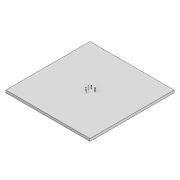
# Autodesk Inventor part: verify_geometry
Saved by Autodesk Inventor 2021 (Build 250183000, 183)
## iProperties
Created: 2022-05-26
Part Number: verify_geometry
Material: Generic
Document SubType Name: Modeling
Designer: Derm
Density: 1 g/cm^3
Appearance: Default
Author: Derm
Autodesk Inventor part; units mm, degrees
ref_plane "YZ Plane" through (0, 0, 0) normal (1, 0, 0) x (0, 1, 0)
ref_plane "XZ Plane" through (0, 0, 0) normal (0, 1, 0) x (-1, 0, 0)
ref_plane "XY Plane" through (0, 0, 0) normal (0, 0, 1) x (1, 0, 0)
sketch "Sketch1" plane through (0, 0, 0) normal (0, 1, 0) x (-1, 0, 0)
  line L0 (-50000, 50000) -> (50000, 50000)
  line L1 (50000, 50000) -> (50000, -50000)
  line L2 (50000, -50000) -> (-50000, -50000)
  line L3 (-50000, -50000) -> (-50000, 50000)
  line L4 (-50000, 50000) -> (50000, -50000) construction
  line L5 (50000, 50000) -> (-50000, -50000) construction
  point P0 (0, 0)
  dimension "d0" = 100000
  dimension "d1" = 100000
  constraints: 12 end point, 2 midpoint, 2 parallel, 1 horizontal, 1 perpendicular
  measures "d0" distance of L0.end L1.end
  measures "d1" distance of L1.end L2.end
extrude "Extrusion1" add sketch "Sketch1" against normal blind 3000
sketch "Sketch2" plane through (0, 0, 0) normal (0, 1, 0) x (1, 0, 0)
  line L0 (50000, 50000) -> (-50000, 50000) projected
  line L1 (-50000, 50000) -> (-50000, -50000) projected
  line L2 (-50000, -50000) -> (50000, -50000) projected
  line L3 (50000, -50000) -> (50000, 50000) projected
  circle A0 centre (-2000, -3000) radius 500
  circle A1 centre (1500, -3000) radius 200
  circle A2 centre (4000, 2000) radius 750
  circle A3 centre (-3000, 1000) radius 200
  circle A4 centre (-1000, 2500) radius 500
  circle A5 centre (600, -5000) radius 250
  point P0 (0, 0)
  dimension "d4" = 1000
  dimension "d5" = 3000
  dimension "d6" = 2000
  dimension "d7" = 400
  dimension "d8" = 3000
  dimension "d9" = 1500
  dimension "d10" = 1500
  dimension "d11" = 2000
  dimension "d13" = 4000
  dimension "d14" = 400
  dimension "d15" = 1000
  dimension "d16" = 3000
  dimension "d17" = 1000
  dimension "d18" = 2500
  dimension "d19" = 1000
  dimension "d20" = 500
  dimension "d21" = 5000
  dimension "d22" = 600
  constraints: 6 centre point
  measures "d4" diameter of A0
  measures "d5" vertical distance of point (0, 0) A0.centre
  measures "d6" horizontal distance of point (0, 0) A0.centre
  measures "d7" diameter of A1
  measures "d8" vertical distance of point (0, 0) A1.centre
  measures "d9" horizontal distance of point (0, 0) A1.centre
  measures "d10" diameter of A2
  measures "d11" vertical distance of point (0, 0) A2.centre
  measures "d13" horizontal distance of A2.centre point (0, 0)
  measures "d14" diameter of A3
  measures "d15" vertical distance of point (0, 0) A3.centre
  measures "d16" horizontal distance of point (0, 0) A3.centre
  measures "d17" diameter of A4
  measures "d18" vertical distance of A4.centre point (0, 0)
  measures "d19" horizontal distance of point (0, 0) A4.centre
  measures "d20" diameter of A5
  measures "d21" vertical distance of point (0, 0) A5.centre
  measures "d22" horizontal distance of point (0, 0) A5.centre
extrude "Extrusion2" add sketch "Sketch2" along normal blind 3000 contours A0 | A1 | A2 | A3 | A4 | A5
body "Solid1"
